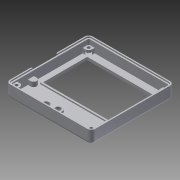
# Autodesk Inventor part: LCDDerivativeTop1
Saved by Autodesk Inventor 2015 SP1 (Build 190203100, 203)
## iProperties
Created: 2015-04-16
Part Number: LCDDerivativeTop1
Material: ABS Plastic
Document SubType Name: Modeling
Designer: Jack
Density: 1.06 g/cm^3
Appearance: Smooth - White
Author: Jack
Autodesk Inventor part; units mm, degrees
ref_plane "YZ Plane" through (0, 0, 0) normal (1, 0, 0) x (0, 1, 0)
ref_plane "XZ Plane" through (0, 0, 0) normal (0, 1, 0) x (-1, 0, 0)
ref_plane "XY Plane" through (0, 0, 0) normal (0, 0, 1) x (1, 0, 0)
sketch "Sketch1" plane through (0, 0, 0) normal (0, 0, 1) x (1, 0, 0)
  line L0 (0, 0) -> (100, 0)
  line L1 (100, 0) -> (100, 97)
  line L2 (100, 97) -> (0, 97)
  line L3 (0, 97) -> (0, 0)
  dimension "d0" = 100
  dimension "d1" = 97
  constraints: 8 end point, 2 parallel, 1 horizontal, 1 perpendicular
  measures "d0" distance of L2.end L1.end
  measures "d1" distance of L1.end L0.end
extrude "Extrusion1" add sketch "Sketch1" along normal blind 2
sketch "Sketch2" plane through (0, 0, 2) normal (0, 0, 1) x (1, 0, 0)
  line L0 (0, 0) -> (100, 0) projected
  line L1 (100, 0) -> (100, 97) projected
  line L2 (100, 97) -> (0, 97) projected
  line L3 (0, 97) -> (0, 0) projected
  line L4 (3, 94) -> (97, 94)
  line L5 (97, 94) -> (97, 3)
  line L6 (97, 3) -> (3, 3)
  line L7 (3, 3) -> (3, 94)
  dimension "d4" = 3
  constraints: 8 end point, 3 other
  measures "d4" distance between parallel lines of L2 L4
extrude "Extrusion2" add sketch "Sketch2" along normal blind 12.9
sketch "Sketch3" plane through (0, 0, 14.9) normal (0, 0, 1) x (1, 0, 0)
  line L0 (97, 94) -> (97, 3) projected
  line L1 (97, 3) -> (3, 3) projected
  line L2 (3, 3) -> (3, 94) projected
  line L3 (3, 94) -> (97, 94) projected
  line L4 (98.6, 95.6) -> (98.6, 1.4)
  line L5 (98.6, 1.4) -> (1.4, 1.4)
  line L6 (1.4, 1.4) -> (1.4, 95.6)
  line L7 (1.4, 95.6) -> (98.6, 95.6)
  dimension "d7" = 1.6
  constraints: 8 end point, 3 other
  measures "d7" distance between parallel lines of L3 L7
extrude "Extrusion3" cut sketch "Sketch3" against normal blind 1.5
sketch "Sketch4" plane through (0, 0, 2) normal (0, 0, 1) x (1, 0, 0)
  line L0 (97, 3) -> (97, 94) projected
  line L1 (97, 94) -> (3, 94) projected
  line L2 (3, 94) -> (3, 3) projected
  arc A0 (10, 6.25) -> (6.25, 10) centre (6.25, 6.25) ccw
  arc A1 (6.25, 87) -> (10, 90.75) centre (6.25, 90.75) ccw
  arc A2 (90, 90.75) -> (93.75, 87) centre (93.75, 90.75) ccw
  arc A3 (93.75, 10) -> (90, 6.25) centre (93.75, 6.25) ccw
  line L3 (10, 6.25) -> (10, 3)
  line L4 (3, 3) -> (97, 3) projected
  line L5 (6.25, 10) -> (3, 10)
  line L6 (10, 90.75) -> (10, 94)
  line L7 (6.25, 87) -> (3, 87)
  line L8 (90, 90.75) -> (90, 94)
  line L9 (93.75, 87) -> (97, 87)
  line L10 (93.75, 10) -> (97, 10)
  line L11 (90, 6.25) -> (90, 3)
  point P0 (0, 0)
  dimension "d32" = 87.5
  dimension "d33" = 3.25
  dimension "d34" = 84.5
  dimension "d35" = 3.25
  dimension "d36" = 7
  constraints: 16 end point, 12 point on line, 8 point on circle, 6 tangent, 5 perpendicular, 4 centre point, 4 coincident, 3 equal radius, 3 vertical alignment, 2 horizontal alignment, 1 vertical
  measures "d32" distance of point (93.75, 6.25) A0.centre
  measures "d33" distance from line of L0 point (93.75, 6.25)
  measures "d34" distance of point (6.25, 6.25) point (6.25, 90.75)
  measures "d35" distance from line of L1 point (6.25, 90.75)
  measures "d36" distance between parallel lines of L1 L9
extrude "Extrusion4" add sketch "Sketch4" along normal blind 5.5 contours L4 L11 A3 L10 L0 | L9 A2 L8 L1 L0 | L4 L2 L5 A0 L3 | L6 A1 L7 L2 L1
sketch "Sketch5" plane through (0, 0, 2) normal (0, 0, 1) x (1, 0, 0)
  line L0 (97, 10) -> (97, 87) projected
  line L1 (10.8, 32.7) -> (89.6, 32.7)
  line L2 (89.6, 32.7) -> (89.6, 84.5)
  line L3 (89.6, 84.5) -> (10.8, 84.5)
  line L4 (10.8, 84.5) -> (10.8, 32.7)
  line L5 (90, 94) -> (10, 94) projected
  point P0 (0, 0)
  dimension "d20" = 51.8
  dimension "d21" = 78.8
  dimension "d22" = 7.4
  dimension "d74" = 9.5
  constraints: 8 end point, 2 parallel, 1 horizontal, 1 perpendicular
  measures "d20" distance of L3.end L1.start
  measures "d21" distance of L1.start L1.end
  measures "d22" distance between parallel lines of L0 L2
  measures "d74" distance between parallel lines of L5 L3
extrude "Extrusion5" cut sketch "Sketch5" against normal up to next
sketch "Sketch6" plane through (0, 0, 2) normal (0, 0, 1) x (1, 0, 0)
  line L0 (89.6, 84.5) -> (89.6, 32.7) projected
  line L1 (89.6, 32.7) -> (10.8, 32.7) projected
  line L2 (10.8, 32.7) -> (10.8, 84.5) projected
  line L3 (10.8, 84.5) -> (89.6, 84.5) projected
  line L4 (91.5, 86.4) -> (91.5, 30.8)
  line L5 (91.5, 30.8) -> (8.9, 30.8)
  line L6 (8.9, 30.8) -> (8.9, 86.4)
  line L7 (8.9, 86.4) -> (91.5, 86.4)
  point P0 (0, 0)
  dimension "d26" = 1.9
  constraints: 8 end point, 3 other
  measures "d26" distance between parallel lines of L3 L7
extrude "Extrusion6" add sketch "Sketch6" along normal blind 1.5
fillet "Fillet1" radius 4.7 4 edges at (0, 97, 7.45) (100, 97, 7.45) (100, 0, 7.45) (0, 0, 7.45)
fillet "Fillet2" radius 3.3 4 edges at (98.6, 1.4, 14.15) (1.4, 1.4, 14.15) (1.4, 95.6, 14.15) (98.6, 95.6, 14.15)
fillet "Fillet3" radius 1.7 4 edges at (3, 3, 10.45) (3, 94, 10.45) (97, 94, 10.45) (97, 3, 10.45)
sketch "Sketch8" plane through (0, 0, 7.5) normal (0, 0, 1) x (1, 0, 0)
  arc A0 (10, 6.25) -> (6.25, 10) centre (6.25, 6.25) ccw projected
  arc A1 (4.7, 94) -> (3, 92.3) centre (4.7, 92.3) ccw projected
  line L0 (3, 87) -> (3, 92.3) projected
  line L1 (3, 87) -> (6.25, 87) projected
  arc A2 (6.25, 87) -> (10, 90.75) centre (6.25, 90.75) ccw projected
  line L2 (10, 90.75) -> (10, 94) projected
  line L3 (4.7, 94) -> (10, 94) projected
  arc A3 (97, 92.3) -> (95.3, 94) centre (95.3, 92.3) ccw projected
  line L4 (90, 94) -> (95.3, 94) projected
  line L5 (90, 94) -> (90, 90.75) projected
  arc A4 (90, 90.75) -> (93.75, 87) centre (93.75, 90.75) ccw projected
  line L6 (93.75, 87) -> (97, 87) projected
  line L7 (97, 92.3) -> (97, 87) projected
  arc A5 (95.3, 3) -> (97, 4.7) centre (95.3, 4.7) ccw projected
  line L8 (97, 10) -> (97, 4.7) projected
  line L9 (97, 10) -> (93.75, 10) projected
  arc A6 (93.75, 10) -> (90, 6.25) centre (93.75, 6.25) ccw projected
  line L10 (90, 6.25) -> (90, 3) projected
  line L11 (95.3, 3) -> (90, 3) projected
  point P0 (0, 0)
hole "Hole2" at (6.25, 90.75, 7.5) at (6.25, 6.25, 7.5) at (93.75, 6.25, 7.5) at (93.75, 90.75, 7.5) direction (0, 0, -1) diameter 3.5 depth 6.5
sketch "Sketch9" plane through (0, 0, 2) normal (0, 0, 1) x (1, 0, 0)
  line L0 (3, 87) -> (3, 10) projected
  arc A0 (10, 6.25) -> (6.25, 10) centre (6.25, 6.25) ccw projected
  arc A1 (93.75, 10) -> (90, 6.25) centre (93.75, 6.25) ccw projected
  line L1 (97, 10) -> (97, 87) projected
  arc A2 (6.25, 22.75) -> (6.25, 29.75) centre (6.25, 26.25) ccw
  arc A3 (93.75, 29.75) -> (93.75, 22.75) centre (93.75, 26.25) ccw
  line L2 (93.75, 29.75) -> (97, 29.75)
  line L3 (97, 4.7) -> (97, 92.3) projected
  line L4 (93.75, 22.75) -> (97, 22.75)
  line L5 (6.25, 29.75) -> (3, 29.75)
  line L6 (6.25, 22.75) -> (3, 22.75)
  point P0 (0, 0)
  dimension "d51" = 20
  dimension "d52" = 7
  dimension "d53" = 7
  constraints: 8 end point, 8 point on line, 4 point on circle, 2 centre point, 2 coincident, 2 perpendicular, 2 tangent, 2 vertical alignment, 1 horizontal alignment
  measures "d51" distance of A1.centre point (93.75, 26.25)
  measures "d52" diameter of A2
  measures "d53" diameter of A3
extrude "Extrusion7" add sketch "Sketch9" along normal blind 5.5
sketch "Sketch11" plane through (0, 0, 2) normal (0, 0, 1) x (1, 0, 0)
  line L0 (97, 87) -> (93.75, 87) projected
  arc A0 (90, 90.75) -> (93.75, 87) centre (93.75, 90.75) ccw projected
  line L1 (90, 94) -> (10, 94) projected
  arc A1 (6.25, 87) -> (10, 90.75) centre (6.25, 90.75) ccw projected
  line L2 (5.4132, 87.627) -> (3.127, 89.9132)
  line L3 (3.127, 89.9132) -> (3.9638, 93.0362)
  line L4 (3.9638, 93.0362) -> (7.0868, 93.873)
  line L5 (7.0868, 93.873) -> (9.373, 91.5868)
  line L6 (5.4132, 87.627) -> (7.5345, 85.5057)
  line L7 (7.5345, 85.5057) -> (11.4943, 89.4655)
  line L8 (11.4943, 89.4655) -> (9.373, 91.5868)
  arc A2 (6.25, 22.75) -> (6.25, 29.75) centre (6.25, 26.25) ccw projected
  line L9 (6.25, 22.75) -> (3, 22.75) projected
  line L10 (3, 22.75) -> (3, 10) projected
  line L11 (3, 10) -> (6.25, 10) projected
  arc A3 (10, 6.25) -> (6.25, 10) centre (6.25, 6.25) ccw projected
  line L12 (10, 6.25) -> (10, 3) projected
  line L13 (10, 3) -> (90, 3) projected
  line L14 (90, 3) -> (90, 6.25) projected
  arc A4 (93.75, 10) -> (90, 6.25) centre (93.75, 6.25) ccw projected
  line L15 (93.75, 10) -> (97, 10) projected
  line L16 (97, 10) -> (97, 22.75) projected
  line L17 (97, 22.75) -> (93.75, 22.75) projected
  arc A5 (93.75, 29.75) -> (93.75, 22.75) centre (93.75, 26.25) ccw projected
  line L18 (91.5, 30.8) -> (8.9, 30.8) projected
  line L19 (8.5362, 8.5362) -> (9.373, 5.4132)
  line L20 (9.373, 5.4132) -> (7.0868, 3.127)
  line L21 (7.0868, 3.127) -> (3.9638, 3.9638)
  line L22 (3.9638, 3.9638) -> (3.127, 7.0868)
  line L23 (3.127, 7.0868) -> (5.4132, 9.373)
  line L24 (5.4132, 9.373) -> (8.5362, 8.5362)
  line L25 (91.4638, 8.5362) -> (94.5868, 9.373)
  line L26 (94.5868, 9.373) -> (96.873, 7.0868)
  line L27 (96.873, 7.0868) -> (96.0362, 3.9638)
  line L28 (96.0362, 3.9638) -> (92.9132, 3.127)
  line L29 (92.9132, 3.127) -> (90.627, 5.4132)
  line L30 (90.627, 5.4132) -> (91.4638, 8.5362)
  line L31 (91.4638, 88.4638) -> (90.627, 91.5868)
  line L32 (90.627, 91.5868) -> (92.9132, 93.873)
  line L33 (92.9132, 93.873) -> (96.0362, 93.0362)
  line L34 (96.0362, 93.0362) -> (96.873, 89.9132)
  line L35 (96.873, 89.9132) -> (94.5868, 87.627)
  line L36 (94.5868, 87.627) -> (91.4638, 88.4638)
  line L37 (5.4132, 9.373) -> (7.5345, 11.4943)
  line L38 (7.5345, 11.4943) -> (11.4943, 7.5345)
  line L39 (11.4943, 7.5345) -> (9.373, 5.4132)
  line L40 (90.627, 91.5868) -> (88.5057, 89.4655)
  line L41 (88.5057, 89.4655) -> (92.4655, 85.5057)
  line L42 (92.4655, 85.5057) -> (94.5868, 87.627)
  line L43 (94.5868, 9.373) -> (92.4655, 11.4943)
  line L44 (92.4655, 11.4943) -> (88.5057, 7.5345)
  line L45 (88.5057, 7.5345) -> (90.627, 5.4132)
  line L46 (3, 29.75) -> (6.25, 29.75) projected
  line L47 (93.75, 29.75) -> (97, 29.75) projected
  line L48 (97, 29.75) -> (97, 87) projected
  line L49 (97, 87) -> (93.75, 87) projected
  arc A6 (90, 90.75) -> (93.75, 87) centre (93.75, 90.75) ccw projected
  line L50 (90, 90.75) -> (90, 94) projected
  line L51 (90, 94) -> (10, 94) projected
  line L52 (10, 94) -> (10, 90.75) projected
  arc A7 (6.25, 87) -> (10, 90.75) centre (6.25, 90.75) ccw projected
  line L53 (6.25, 87) -> (3, 87) projected
  line L54 (3, 87) -> (3, 29.75) projected
  line L55 (8.9, 30.8) -> (8.9, 86.4) projected
  line L56 (8.9, 86.4) -> (91.5, 86.4) projected
  line L57 (91.5, 86.4) -> (91.5, 30.8) projected
  point P0 (0, 0)
  dimension "d63" = 5.6
  dimension "d64" = 45
  dimension "d65" = 3
  dimension "d66" = 45
  dimension "d67" = 3
  dimension "d68" = 45
  dimension "d69" = 45
  dimension "d70" = 3
  dimension "d71" = 3
  constraints: 68 end point, 7 perpendicular, 5 collinear, 4 coincident, 3 equal length, 47 other
  measures "d63" distance between parallel lines of L2 L5
  measures "d64" angle of L1 L5
  measures "d65" distance of L7.end L5.end
  measures "d66" angle of L13 L20
  measures "d67" distance of L38.end L19.end
  measures "d68" angle of L13 L29
  measures "d69" angle of L0 L35
  measures "d70" distance of L31.end L40.end
  measures "d71" distance of L25.end L43.end
extrude "Extrusion8" cut sketch "Sketch11" along normal blind 3 contours L42 L41 L40 L50 A0 L0 | L0 A0 L50 L40 L31 L36 L42 | L36 L31 L32 L33 L34 L35 | L43 L25 L30 L45 L14 A4 L15 | L15 A4 L14 L45 L44 L43 | L52 A1 L53 L6 L2 L3 L4 L5 L8 | L8 L7 L6 L53 A1 L52 | L26 L27 L28 L29 L30 L25 | L39 L19 L24 L37 L11 A3 L12 | L12 A3 L11 L37 L38 L39 | L20 L21 L22 L23 L24 L19
sketch "Sketch12" plane through (0, 0, 7.5) normal (0, 0, 1) x (1, 0, 0)
  circle A0 centre (6.25, 6.25) radius 1.75 projected
  arc A1 (3, 4.7) -> (4.7, 3) centre (4.7, 4.7) ccw projected
  line L0 (10, 3) -> (4.7, 3) projected
  line L1 (10, 3) -> (10, 6.25) projected
  arc A2 (10, 6.25) -> (6.25, 10) centre (6.25, 6.25) ccw projected
  line L2 (6.25, 10) -> (3, 10) projected
  line L3 (3, 4.7) -> (3, 10) projected
  circle A3 centre (93.75, 6.25) radius 1.75 projected
  arc A4 (95.3, 3) -> (97, 4.7) centre (95.3, 4.7) ccw projected
  line L4 (97, 10) -> (97, 4.7) projected
  line L5 (97, 10) -> (93.75, 10) projected
  arc A5 (93.75, 10) -> (90, 6.25) centre (93.75, 6.25) ccw projected
  line L6 (90, 6.25) -> (90, 3) projected
  line L7 (95.3, 3) -> (90, 3) projected
  point P0 (0, 0)
extrude "Extrusion9" add sketch "Sketch12" along normal blind 4.25
sketch "Sketch13" plane through (0, 4.7, 0) normal (-1, 0, 0) x (0, 0, 1)
  line L0 (14.9, 0) -> (0, 0) projected
  line L1 (14.9, 87.6) -> (14.9, 0) projected
  line L2 (0, 87.6) -> (14.9, 87.6) projected
  line L3 (14.9, 87.6) -> (14.9, 0) projected
  line L4 (14.9, 53.4) -> (13.4, 53.4)
  line L5 (13.4, 53.4) -> (13.4, 25.7)
  line L6 (13.4, 87.6) -> (13.4, 0) projected
  line L7 (13.4, 25.7) -> (14.9, 25.7)
  point P0 (0, -4.7)
  dimension "d77" = 1.5
  dimension "d78" = 34.2
  dimension "d79" = 25.7
  constraints: 6 end point, 3 point on line, 2 perpendicular
  measures "d77" distance of L4.start L4.end
  measures "d78" distance between parallel lines of L2 L4
  measures "d79" distance between parallel lines of L0 L7
extrude "Extrusion10" cut sketch "Sketch13" against normal up to surface (1.4 mm away) contours L7 L5 L4 L1
chamfer "Chamfer1" distance 1.4 angle 45 3 edges at (0, 30.4, 14.15) (0, 44.25, 13.4) (0, 58.1, 14.15)
sketch "Sketch14" plane through (0, 0, 0) normal (0, 0, -1) x (-1, 0, 0)
  line L0 (0, 92.3) -> (0, 4.7) projected
  line L1 (-4.7, 0) -> (-95.3, 0) projected
  circle A0 centre (-33.05, 13.9) radius 3.75
  point P0 (0, 0)
  dimension "d86" = 7.5
  dimension "d87" = 33.05
  dimension "d88" = 13.9
  constraints: 1 centre point
  measures "d86" diameter of A0
  measures "d87" distance from line of L0 A0.centre
  measures "d88" distance from line of L1 A0.centre
extrude "Extrusion11" cut sketch "Sketch14" against normal up to next
sketch "Sketch15" plane through (0, 0, 0) normal (0, 0, -1) x (-1, 0, 0)
  line L0 (0, 92.3) -> (0, 4.7) projected
  line L1 (-4.7, 0) -> (-95.3, 0) projected
  line L2 (-47.3, 8.95) -> (-47.3, 14.05) construction
  line L3 (-44.4, 8.95) -> (-44.4, 14.05)
  line L4 (-50.2, 14.05) -> (-50.2, 8.95)
  arc A0 (-50.2, 8.95) -> (-44.4, 8.95) centre (-47.3, 8.95) ccw
  arc A1 (-44.4, 14.05) -> (-50.2, 14.05) centre (-47.3, 14.05) ccw
  point P0 (0, 0)
  point P1 (-47.3, 11.5)
  dimension "d91" = 2.55
  dimension "d92" = 5.8
  dimension "d93" = 47.3
  dimension "d94" = 11.5
  constraints: 8 end point, 4 point on circle, 4 tangent, 2 centre point, 1 midpoint, 1 parallel, 1 vertical
  measures "d91" distance of point (-47.3, 11.5) L2.end
  measures "d92" diameter of A1
  measures "d93" distance from line of L0 point (-47.3, 11.5)
  measures "d94" distance from line of L1 point (-47.3, 11.5)
extrude "Extrusion12" cut sketch "Sketch15" against normal up to next
sketch "Sketch16" plane through (0, 0, 2) normal (0, 0, 1) x (1, 0, 0)
  arc A0 (50.2, 14.05) -> (44.4, 14.05) centre (47.3, 14.05) ccw projected
  line L0 (50.2, 14.05) -> (50.2, 8.95) projected
  arc A1 (44.4, 8.95) -> (50.2, 8.95) centre (47.3, 8.95) ccw projected
  line L1 (44.4, 8.95) -> (44.4, 14.05) projected
  line L2 (52.2, 8.95) -> (52.2, 14.05)
  arc A2 (52.2, 14.05) -> (42.4, 14.05) centre (47.3, 14.05) ccw
  line L3 (42.4, 14.05) -> (42.4, 8.95)
  arc A3 (42.4, 8.95) -> (52.2, 8.95) centre (47.3, 8.95) ccw
  point P0 (0, 0)
  dimension "d97" = 2
  constraints: 4 end point, 4 point on circle, 2 centre point, 3 other
  measures "d97" distance between parallel lines of L0 L2
extrude "Extrusion13" add sketch "Sketch16" along normal blind 2.4
chamfer "Chamfer3" distance 1.5 angle 45 4 edges at (47.3, 6.05, 0) (50.2, 11.5, 0) (47.3, 16.95, 0) (44.4, 11.5, 0)
fillet "Fillet4" radius 3 8 edges at (98.6234, 95.6234, 0) (50, 97, 0) (1.3766, 95.6234, 0) (0, 48.5, 0) (1.3766, 1.3766, 0) (50, 0, 0) (98.6234, 1.3766, 0) (100, 48.5, 0)
body "Solid1"
